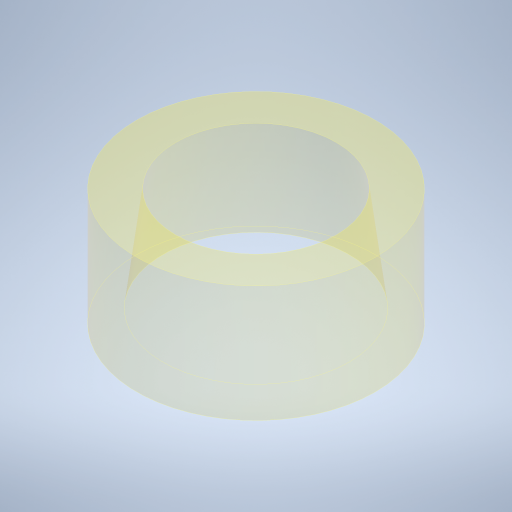
# Autodesk Inventor part: Gripper
Saved by Autodesk Inventor 2024 (Build 280153000, 153)
## iProperties
Created: 2023-12-19
Part Number: Gripper
Material: Thermoplastic Resin
Document SubType Name: Modeling
Designer: greg
Density: 1.28 g/cm^3
Appearance: Clear - Yellow
Author: greg
Autodesk Inventor part; units mm, degrees
ref_plane "YZ Plane" through (0, 0, 0) normal (1, 0, 0) x (0, 1, 0)
ref_plane "XZ Plane" through (0, 0, 0) normal (0, 1, 0) x (-1, 0, 0)
ref_plane "XY Plane" through (0, 0, 0) normal (0, 0, 1) x (1, 0, 0)
sketch "Sketch1" plane through (0, 0, 0) normal (0, 0, 1) x (1, 0, 0)
  line L0 (0, 0) -> (0, 14.2875)
  line L1 (0, 14.2875) -> (9.8425, 14.2875) construction
  line L2 (9.8425, 14.2875) -> (14.605, 14.2875)
  line L3 (14.605, 14.2875) -> (14.605, 0)
  line L4 (14.605, 0) -> (11.43, 1.5875)
  line L5 (11.43, 1.5875) -> (9.8425, 14.2875)
  dimension "d1" = 19.685
  dimension "d2" = 1.5875
  dimension "d3" = 3.175
  dimension "d5" = 14.2875
  dimension "d6" = 12.7
  constraints: 12 end point, 1 horizontal, 1 horizontal alignment, 1 perpendicular, 1 point on line, 1 vertical
  measures "d1" diameter of L1.end L0
  measures "d2" horizontal distance of L1.end L4.end
  measures "d3" horizontal distance of L3.end L4.end
  measures "d5" distance of L2.end L3.end
  measures "d6" vertical distance of L4.end L1.end
revolve "Revolution1" add sketch "Sketch1" angle 360 about axis through (0, 0, 0) along (0, 1, 0)
body "Solid1"
